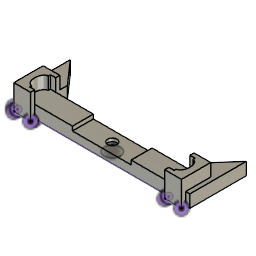
Servo Horn Topper (Autodesk Fusion 360 design; units mm, degrees)
Autodesk Fusion 360 part; units mm, degrees
sketch "Sketch1" plane through (0, 0, 0) normal (0, 0, 1) x (1, 0, 0)
  line L0 (-7, 1.5) -> (35, 1.5)
  line L1 (35, 1.5) -> (35, -3.5)
  line L2 (35, -3.5) -> (-7, -3.5)
  line L3 (-7, -3.5) -> (-7, 1.5)
  line L4 (-7, 1.5) -> (-7, 10)
  line L5 (-7, 10) -> (-2, 4.3)
  line L6 (-2, 4.3) -> (-2, 1.5)
  line L7 (35, 1.5) -> (35, 10)
  line L8 (35, 10) -> (30, 4.3)
  line L9 (30, 4.3) -> (30, 1.5)
  dimension "d1" = 5
  dimension "d2" = 42
  dimension "d13" = 8.5
  dimension "d14" = 5
  dimension "d15" = 2.8
  constraint horizontal L0
  constraint vertical L1
  constraint horizontal L2
  constraint vertical L3
  constraint perpendicular L0 L4
  constraint coincident L0 L6.end
  constraint perpendicular L0 L6
  constraint perpendicular L0 L7
  constraint coincident L0 L9.end
  constraint perpendicular L0 L9
  constraint equal L4 L7
  constraint equal L6 L9
  constraint equal L5 L8
  measures "d1" distance of L0.start L2.end
  measures "d2" distance of L0.start L0.end
  measures "d13" distance of L0.start L4.end
  measures "d14" distance of L4 L6
  measures "d15" distance of L5.end L6.end
extrude "Extrude1" add sketch "Sketch1" along normal blind 3
sketch "Sketch2" plane through (0, 0, 3) normal (0, 0, 1) x (-1, 0, 0)
  line L0 (-35, 3.5) -> (-35, -10)
  line L1 (-35, -10) -> (-30, -4.3)
  line L2 (-30, -4.3) -> (-30, -1.5)
  line L3 (-30, -1.5) -> (2, -1.5)
  line L4 (2, -1.5) -> (2, -4.3)
  line L5 (2, -4.3) -> (7, -10)
  line L6 (7, -10) -> (7, 3.5)
  line L7 (7, 3.5) -> (-35, 3.5)
  line L8 (-7, -1.5) -> (-21, -1.5)
  line L9 (-21, -1.5) -> (-21, 3.5)
  line L10 (-21, 3.5) -> (-7, 3.5)
  line L11 (-7, 3.5) -> (-7, -1.5)
  line L12 (-7, -1.5) -> (-21, 3.5) construction
  line L13 (-21, -1.5) -> (-7, 3.5) construction
  point P0 (-14, 1)
  dimension "d16" = 14
  dimension "d17" = 14
  dimension "d18" = 5
  constraint horizontal L8
  constraint perpendicular L8 L9
  constraint parallel L8 L10
  constraint parallel L9 L11
  constraint coincident L12 P0
  constraint coincident L13 P0
  constraint coincident L3 L8.start
  measures "d16" distance of L0 L9
  measures "d17" distance of L6 L11
  measures "d18" distance of L8.end L9.end
extrude "Extrude2" cut sketch "Sketch2" against normal blind 1 contours L3 L7 L8 L9 L10 L11
sketch "Sketch3" plane through (0, 0, 3) normal (0, 0, 1) x (-1, 0, 0)
  line L0 (-21, -1.5) -> (-21, 3.5)
  line L1 (-21, 3.5) -> (-35, 3.5)
  line L2 (-35, 3.5) -> (-35, -10)
  line L3 (-35, -10) -> (-30, -4.3)
  line L4 (-30, -4.3) -> (-30, -1.5)
  line L5 (-30, -1.5) -> (-21, -1.5)
  line L6 (6, -1.5) -> (-34, -1.5)
  line L7 (-34, -1.5) -> (-34, 3.5)
  line L8 (-34, 3.5) -> (6, 3.5)
  line L9 (6, 3.5) -> (6, -1.5)
  line L10 (6, -1.5) -> (-34, 3.5) construction
  line L11 (-34, -1.5) -> (6, 3.5) construction
  ellipse E0 centre (3.25, 1) end of major axis (4.5, 1) minor radius 2
  line L12 (2, 1) -> (4.5, 1) construction
  line L13 (3.25, -1) -> (3.25, 3) construction
  line L14 (3.2507, 3.5) -> (3.25, 3)
  line L15 (3.25, -1) -> (3.25, -1.5)
  ellipse E1 centre (-31.25, 0.9902) end of major axis (-32.5, 0.9902) minor radius 2
  line L16 (-30, 0.9902) -> (-32.5, 0.9902) construction
  line L17 (-31.25, 2.9902) -> (-31.25, -1.0098) construction
  line L18 (-31.25, 2.9902) -> (-31.25, 3.5)
  line L19 (-31.25, -1.5) -> (-31.25, -1.0098)
  line L20 (6, -2.5) -> (2, -2.5)
  line L21 (2, -2.5) -> (2, -1.5)
  line L22 (2, -1.5) -> (6, -1.5)
  line L23 (6, -1.5) -> (6, -2.5)
  line L24 (-34, -1.5) -> (-30, -1.5)
  line L25 (-30, -1.5) -> (-30, -2.5)
  line L26 (-30, -2.5) -> (-34, -2.5)
  line L27 (-34, -2.5) -> (-34, -1.5)
  point P0 (-14, 1)
  dimension "d7" = 40
  dimension "d8" = 2.5
  dimension "d9" = 4
  dimension "d10" = 2.5
  dimension "d19" = 5
  dimension "d20" = 21
  dimension "d21" = 2.5
  dimension "d22" = 37
  dimension "d23" = 1.5
  dimension "d24" = 5
  constraint horizontal L6
  constraint perpendicular L6 L7
  constraint parallel L6 L8
  constraint parallel L7 L9
  constraint coincident L10 P0
  constraint coincident L11 P0
  constraint coincident E0 L12.start
  constraint coincident E0 L12.end
  constraint coincident E0 L13.start
  constraint coincident E0 L13.end
  constraint perpendicular L9 L12
  constraint coincident L8 L14.start
  constraint coincident L13.end L14.end
  constraint coincident L13.start L15.start
  constraint coincident L6 L15.end
  constraint perpendicular L6 L15
  constraint coincident E1 L16.start
  constraint coincident E1 L16.end
  constraint coincident E1 L17.start
  constraint coincident E1 L17.end
  constraint perpendicular L7 L16
  constraint coincident L17.start L18.start
  constraint coincident L8 L18.end
  constraint perpendicular L8 L18
  constraint coincident L6 L19.start
  constraint coincident L17.end L19.end
  constraint perpendicular L6 L19
  constraint horizontal L20
  constraint vertical L21
  constraint horizontal L22
  constraint vertical L23
  constraint coincident L6 L21.end
  constraint horizontal L24
  constraint vertical L25
  constraint horizontal L26
  constraint vertical L27
  constraint coincident L4 L25.end
  measures "d7" distance of L7.end L8.end
  measures "d8" distance of E0
  measures "d10" distance of E1
  measures "d19" distance of L6.start L8.end
  measures "d20" distance of L2 P0
  measures "d21" distance of L8 E0.centre
  measures "d22" horizontal distance of L12.end L16.end
  measures "d23" distance of L9 L12.end
  measures "d24" distance of L1 L6
extrude "Extrude3" add sketch "Sketch3" along normal blind 3 contours L4 L6 L24 L25 L26 L27 | L6 L20 L21 L22 L23 | L1 L6 L7 L8 E1 L18 L19 L24 | L6 L8 L9 E0 L14 L15 L22
sketch "Sketch6" plane through (0, -3.5, 0) normal (0, -1, 0) x (1, 0, 0)
  line L0 (21, 3) -> (21, 2)
  line L1 (21, 2) -> (7, 2)
  line L2 (7, 2) -> (7, 3)
  line L3 (7, 3) -> (-3.2507, 3)
  line L4 (-3.2507, 3) -> (-3.2507, 6)
  line L5 (-3.2507, 6) -> (-6, 6)
  line L6 (-6, 6) -> (-6, 3)
  line L7 (-6, 3) -> (-7, 3)
  line L8 (-7, 3) -> (-7, 0)
  line L9 (-7, 0) -> (35, 0)
  line L10 (35, 0) -> (35, 3)
  line L11 (35, 3) -> (34, 3)
  line L12 (34, 3) -> (34, 6)
  line L13 (34, 6) -> (31.25, 6)
  line L14 (31.25, 6) -> (31.25, 3)
  line L15 (31.25, 3) -> (21, 3)
  line L16 (-2, 6) -> (-6, 6)
  line L17 (-6, 6) -> (-6, 0)
  line L18 (-6, 0) -> (-2, 0)
  line L19 (-2, 0) -> (-2, 6)
  line L20 (34, 6) -> (30, 6)
  line L21 (30, 6) -> (30, 0)
  line L22 (30, 0) -> (34, 0)
  line L23 (34, 0) -> (34, 6)
  constraint horizontal L16
  constraint vertical L17
  constraint horizontal L18
  constraint vertical L19
  constraint coincident L9 L17.end
  constraint horizontal L20
  constraint vertical L21
  constraint horizontal L22
  constraint vertical L23
  constraint coincident L9 L21.end
  constraint coincident L12.end L13.start
extrude "Extrude6" add sketch "Sketch6" along normal blind 1 contours L14 L15 L20 L21 | L9 L12 L13 L14 L15 L20 L21 L22 L23 | L3 L4 L5 L6 L9 L16 L17 L18 L19 | L3 L4 L16 L19
sketch "Sketch4" plane through (0, 0, 0) normal (0, 0, -1) x (1, 0, 0)
  line L0 (35, -10) -> (35, 3.5)
  line L1 (35, 3.5) -> (34, 3.5)
  line L2 (-7, 3.5) -> (-7, -10)
  line L3 (-7, -10) -> (-2, -4.3)
  line L4 (-2, -4.3) -> (-2, -1.5)
  line L5 (-2, -1.5) -> (30, -1.5)
  line L6 (30, -1.5) -> (30, -4.3)
  line L7 (30, -4.3) -> (35, -10)
  line L8 (5, 3.5) -> (23, 3.5)
  line L9 (23, 3.5) -> (23, -1.5)
  line L10 (23, -1.5) -> (5, -1.5)
  line L11 (5, -1.5) -> (5, 3.5)
  circle A0 centre (14, 1) radius 1.125
  line L12 (34, 3.5) -> (34, 4.5)
  line L13 (34, 4.5) -> (30, 4.5)
  line L14 (30, 4.5) -> (30, 3.5)
  line L15 (30, 3.5) -> (-2, 3.5)
  line L16 (-2, 3.5) -> (-2, 4.5)
  line L17 (-2, 4.5) -> (-6, 4.5)
  line L18 (-6, 4.5) -> (-6, 3.5)
  line L19 (-6, 3.5) -> (-7, 3.5)
  dimension "d25" = 2.25
  constraint horizontal L8
  constraint vertical L9
  constraint horizontal L10
  constraint vertical L11
  constraint coincident L5 L9.end
  constraint coincident L1 L8.start
  measures "d25" diameter of A0
extrude "Extrude4" cut sketch "Sketch4" against normal blind 2 contours A0
sketch "Sketch5" plane through (0, 0, 0) normal (0, 0, -1) x (1, 0, 0)
  circle A0 centre (14, 1) radius 1.125
  line L0 (35, -10) -> (35, 3.5)
  line L1 (35, 3.5) -> (34, 3.5)
  line L2 (-7, 3.5) -> (-7, -10)
  line L3 (-7, -10) -> (-2, -4.3)
  line L4 (-2, -4.3) -> (-2, -1.5)
  line L5 (-2, -1.5) -> (30, -1.5)
  line L6 (30, -1.5) -> (30, -4.3)
  line L7 (30, -4.3) -> (35, -10)
  circle A1 centre (14, 1) radius 1.875
  line L8 (34, 3.5) -> (34, 4.5)
  line L9 (34, 4.5) -> (30, 4.5)
  line L10 (30, 4.5) -> (30, 3.5)
  line L11 (30, 3.5) -> (-2, 3.5)
  line L12 (-2, 3.5) -> (-2, 4.5)
  line L13 (-2, 4.5) -> (-6, 4.5)
  line L14 (-6, 4.5) -> (-6, 3.5)
  line L15 (-6, 3.5) -> (-7, 3.5)
  dimension "d28" = 3.75
  constraint concentric A0 A1
  measures "d28" diameter of A1
extrude "Extrude5" cut sketch "Sketch5" against normal blind 1.25 contours A1
equation "d16 = d17"
equation "d18 = d1"
equation "d19 = d1"
equation "d20 = d2 / 2"
equation "d21 = d1 / 2"
equation "d24 = d1"
